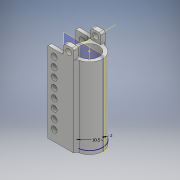
# Autodesk Inventor part: magnet-holder
Saved by Autodesk Inventor 2018 (Build 220112000, 112)
## iProperties
Created: 2025-03-11
Part Number: magnet-holder
Material: Generic
Document SubType Name: Modeling
Designer: neo
Density: 1 g/cm^3
Appearance: Default
Author: neo
Autodesk Inventor part; units mm, degrees
ref_plane "YZ Plane" through (0, 0, 0) normal (1, 0, 0) x (0, 1, 0)
ref_plane "XZ Plane" through (0, 0, 0) normal (0, 1, 0) x (-1, 0, 0)
ref_plane "XY Plane" through (0, 0, 0) normal (0, 0, 1) x (1, 0, 0)
sketch "Sketch1" plane through (0, 0, 0) normal (0, 0, 1) x (1, 0, 0)
  circle A0 centre (0, 0) radius 5.25
  circle A1 centre (0, 0) radius 7.25
  dimension "d0" = 10.5
  dimension "d1" = 2
  constraints: 2 centre point, 2 coincident
  measures "d0" diameter of A0
  measures "d1" radial gap between concentric circles of A0 A1
extrude "Extrusion1" add sketch "Sketch1" along normal blind 42.5
extrude "Extrusion2" add sketch "Sketch1" against normal blind 2 contours A0 | A1
sketch "Sketch2" plane through (0, 0, -2) normal (0, 0, -1) x (-1, 0, 0)
  circle A0 centre (0, 0) radius 7.25 construction
  circle A1 centre (0, 0) radius 3.5
  dimension "d6" = 7
  constraints: 1 centre point, 1 coincident
  measures "d6" diameter of A1
extrude "Extrusion3" cut sketch "Sketch2" against normal through all
sketch "Sketch3" plane through (0, 0, 42.5) normal (0, 0, 1) x (1, 0, 0)
  circle A0 centre (0, 0) radius 7.25 construction
  circle A1 centre (0, 0) radius 5.25 construction
  line L0 (0, 0) -> (-18.4312, 0) construction
  circle A2 centre (0, 0) radius 7.25 construction
  line L1 (-2.6458, 6.75) -> (-14.25, 6.75) construction
  line L2 (-14.25, 6.75) -> (-14.25, -6.75) construction
  line L3 (-14.25, -6.75) -> (-2.6458, -6.75) construction
  line L4 (-2.6458, -6.75) -> (-2.6458, 6.75) construction
  line L5 (-7.25, 0) -> (-7.25, 11.3017) construction
  line L6 (-14.25, 6.75) -> (0, 6.75)
  line L7 (0, 6.75) -> (0, 8.75)
  line L8 (0, 8.75) -> (-14.25, 8.75)
  line L9 (-14.25, 8.75) -> (-14.25, 6.75)
  dimension "d9" = 7
  dimension "d10" = 13.5
  dimension "d11" = 2
  dimension "d16" = 0
  constraints: 20 end point, 4 parallel, 3 horizontal, 3 perpendicular, 2 point on circle, 1 point on line, 1 tangent, 1 vertical, 3 other
  measures "d9" distance between parallel lines of L2 L5
  measures "d10" distance of L1.end L2.end
  measures "d11" distance of L8.end L1.end
  measures "d16" distance from line of point (0, 0) L7
extrude "Extrusion4" add sketch "Sketch3" against normal up to surface (44.5 mm away)
ref_plane "Work Plane1" through (0, 0, 42.5) normal (0, 1, 0) x (1, 0, 0)
mirror "Mirror1" about plane through (0, 0, 42.5) normal (0, 1, 0) of "Extrusion4"
fillet "Fillet1" radius 2 2 edges at (0, 7.25, 20.25) (0, -7.25, 20.25)
fillet "Fillet2" radius 2 2 edges at (-2.6458, 6.75, 20.25) (-2.6458, -6.75, 20.25)
sketch "Sketch4" plane through (-14.25, -8.75, -2) normal (0, -1, 0) x (1, 0, 0)
  line L0 (0, 0) -> (14.25, 0) construction
  line L1 (14.25, 44.5) -> (14.25, 0) construction
  line L2 (14.25, 44.5) -> (0, 44.5) construction
  line L3 (0, 44.5) -> (0, 0) construction
  line L4 (3.5, 56.7252) -> (3.5, -16.7448) construction
  circle A0 centre (3.5, 6) radius 1.6
  line L5 (3.5, 61.7252) -> (3.5, -11.7448) construction
  circle A1 centre (3.5, 11) radius 1.6
  line L6 (3.5, 66.7252) -> (3.5, -6.7448) construction
  circle A2 centre (3.5, 16) radius 1.6
  line L7 (3.5, 71.7252) -> (3.5, -1.7448) construction
  circle A3 centre (3.5, 21) radius 1.6
  line L8 (3.5, 76.7252) -> (3.5, 3.2552) construction
  circle A4 centre (3.5, 26) radius 1.6
  line L9 (3.5, 81.7252) -> (3.5, 8.2552) construction
  circle A5 centre (3.5, 31) radius 1.6
  line L10 (3.5, 86.7252) -> (3.5, 13.2552) construction
  circle A6 centre (3.5, 36) radius 1.6
  line L11 (3.5, 91.7252) -> (3.5, 18.2552) construction
  circle A7 centre (3.5, 41) radius 1.6
  point P0 (14.25, 2)
  dimension "d19" = 3.5
  dimension "d20" = 3.2
  dimension "d21" = 6
  dimension "d24" = 5
  constraints: 16 end point, 8 centre point, 8 point on line, 2 vertical, 35 other
  measures "d19" distance between parallel lines of L3 L4
  measures "d20" diameter of A0
  measures "d21" distance from line of L0 A0.centre
  measures "d24" distance of L4.start L5.start
extrude "Extrusion5" cut sketch "Sketch4" against normal through all
sketch "Sketch5" plane through (0, 0, 42.5) normal (0, 0, 1) x (1, 0, 0)
  arc A0 (1.5515, -7.082) -> (1.5515, 7.082) centre (0, 0) ccw construction
  arc A1 (0, 8.75) -> (1.5515, 7.082) centre (1.9795, 9.0357) ccw construction
  line L0 (0, 8.75) -> (-14.25, 8.75) construction
  line L1 (-14.25, 8.75) -> (-14.25, 6.75) construction
  line L2 (-14.25, 6.75) -> (-7.9373, 6.75) construction
  arc A2 (-6.2211, 3.723) -> (-7.9373, 6.75) centre (-7.9373, 4.75) ccw construction
  arc A3 (-6.2211, 3.723) -> (-6.2211, -3.723) centre (0, 0) ccw construction
  arc A4 (-7.9373, -6.75) -> (-6.2211, -3.723) centre (-7.9373, -4.75) ccw construction
  line L3 (-14.25, -6.75) -> (-7.9373, -6.75) construction
  line L4 (-14.25, -8.75) -> (-14.25, -6.75) construction
  line L5 (0, -8.75) -> (-14.25, -8.75) construction
  arc A5 (1.5515, -7.082) -> (0, -8.75) centre (1.9795, -9.0357) ccw construction
  circle A6 centre (0, 0) radius 5.25 construction
  line L6 (0, 8.75) -> (-14.25, 8.75) projected
  line L7 (0, 8.75) -> (-5.5, 8.75)
  line L8 (-5.5, 8.75) -> (-5.5, 6.25)
  line L9 (-5.5, 6.25) -> (0, 6.25)
  line L10 (0, 6.25) -> (0, 8.75)
  dimension "d31" = 2.5
  dimension "d32" = 5.5
  constraints: 8 end point, 2 parallel, 1 horizontal, 1 perpendicular
  measures "d31" distance of L9.end L0.start
  measures "d32" distance of L8.end L9.end
extrude "Extrusion6" add sketch "Sketch5" along normal blind 5.5
mirror "Mirror2" about plane through (0, 0, 42.5) normal (0, 1, 0) of "Extrusion6"
sketch "Sketch6" plane through (-14.25, 8.75, 42.5) normal (0, 1, 0) x (1, 0, 0)
  circle A0 centre (3.5, 8.5) radius 1.6 construction
  circle A1 centre (3.5, 18.5) radius 1.6 construction
  circle A2 centre (3.5, 28.5) radius 1.6 construction
  circle A3 centre (3.5, 38.5) radius 1.6 construction
  circle A4 centre (3.5, 33.5) radius 1.6 construction
  circle A5 centre (3.5, 23.5) radius 1.6 construction
  circle A6 centre (3.5, 13.5) radius 1.6 construction
  circle A7 centre (3.5, 3.5) radius 1.6 construction
  line L0 (0, 44.5) -> (14.25, 44.5) construction
  line L1 (0, 0) -> (0, 44.5) construction
  line L2 (8.75, 0) -> (0, 0) construction
  line L3 (8.75, 0) -> (8.75, -5.5) construction
  line L4 (14.25, -5.5) -> (8.75, -5.5) construction
  line L5 (14.25, 0) -> (14.25, -5.5) construction
  line L6 (14.25, 0) -> (14.25, 44.5) construction
  line L7 (14.25, 0) -> (14.25, 44.5) construction
  line L8 (14.25, 0) -> (8.75, -5.5) construction
  line L9 (8.75, -5.5) -> (14.25, -5.5) construction
  line L10 (14.25, -5.5) -> (8.75, 0) construction
  circle A8 centre (11.5, -2.75) radius 1.6
  point P0 (14.25, 42.5)
  dimension "d35" = 3.2
  constraints: 4 end point, 1 centre point, 1 midpoint, 1 perpendicular
  measures "d35" diameter of A8
extrude "Extrusion7" cut sketch "Sketch6" against normal through all
fillet "Fillet3" radius 1 6 edges at (-5.5, 7.5, 42.5) (-5.5, 7.5, 48) (0, 7.5, 48) (-5.5, -7.5, 42.5) (-5.5, -7.5, 48) (0, -7.5, 48)
body "Solid1"
